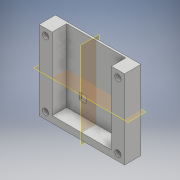
# Autodesk Inventor part: Case_Top_Partv1
Saved by Autodesk Inventor 2017 (Build 210142000, 142)
## iProperties
Created: 2020-01-23
Part Number: Case_Top_Partv1
Material: Generic
Document SubType Name: Modeling
Designer: Manny
Density: 1 g/cm^3
Appearance: Default
Author: Manny
Autodesk Inventor part; units mm, degrees
ref_plane "YZ Plane" through (0, 0, 0) normal (1, 0, 0) x (0, 1, 0)
ref_plane "XZ Plane" through (0, 0, 0) normal (0, 1, 0) x (-1, 0, 0)
ref_plane "XY Plane" through (0, 0, 0) normal (0, 0, 1) x (1, 0, 0)
sketch "Sketch1" plane through (0, 0, 0) normal (0, 1, 0) x (-1, 0, 0)
  line L0 (0, 0) -> (-130, 0)
  line L1 (-130, 0) -> (-130, -120)
  line L2 (-130, -120) -> (0, -120)
  line L3 (0, -120) -> (0, 0)
  dimension "d0" = 130
  dimension "d1" = 120
  constraints: 8 end point, 2 parallel, 1 horizontal, 1 perpendicular
  measures "d0" distance of L1.end L2.end
  measures "d1" distance of L0.end L1.end
extrude "Extrusion1" add sketch "Sketch1" along normal blind 25
sketch "Sketch2" plane through (0, 0, 0) normal (0, -1, 0) x (1, 0, 0)
  line L0 (110, -6.6572) -> (20, -6.6572)
  line L1 (20, -6.6572) -> (20, -110)
  line L2 (20, -110) -> (110, -110)
  line L3 (110, -110) -> (110, -6.6572)
  line L4 (0, -120) -> (0, 0) projected
  line L5 (0, 0) -> (130, 0) projected
  line L6 (130, -120) -> (0, -120) projected
  line L7 (130, 0) -> (130, -120) projected
  dimension "d5" = 6.6572
  dimension "d46" = 20
  dimension "d47" = 20
  dimension "d48" = 10
  constraints: 8 end point, 2 parallel, 1 horizontal, 1 perpendicular
  measures "d5" distance between parallel lines of L5 L0
  measures "d46" distance between parallel lines of L4 L1
  measures "d47" distance between parallel lines of L7 L3
  measures "d48" distance between parallel lines of L2 L6
extrude "Extrusion2" cut sketch "Sketch2" against normal blind 22 contours L3 L2 L1 L0
sketch "Sketch4" plane through (0, 22, 0) normal (0, -1, 0) x (1, 0, 0)
  line L0 (130, -120) -> (0, -120) projected
  line L1 (40, -90) -> (50, -90)
  line L2 (50, -90) -> (50, -80)
  line L3 (50, -80) -> (40, -80)
  line L4 (40, -80) -> (40, -90)
  line L5 (0, -120) -> (0, 0) projected
  line L6 (20, -110) -> (20, -6.6572) projected
  line L7 (110, -110) -> (20, -110) projected
  dimension "d42" = 10
  dimension "d43" = 10
  dimension "d49" = 20
  dimension "d50" = 20
  constraints: 8 end point, 2 parallel, 1 horizontal, 1 perpendicular
  measures "d42" distance of L1.start L1.end
  measures "d43" distance of L3.end L1.start
  measures "d49" distance between parallel lines of L4 L6
  measures "d50" distance between parallel lines of L1 L7
extrude "Extrusion3" cut sketch "Sketch4" against normal blind 22
sketch "Sketch5" plane through (0, 0, 0) normal (0, 0, 1) x (1, 0, 0)
  line L0 (20, 22) -> (110, 22)
  line L1 (110, 22) -> (110, 0)
  line L2 (110, 0) -> (20, 0)
  line L3 (20, 0) -> (20, 22)
  line L4 (0, 0) -> (0, 25) projected
  line L5 (130, 0) -> (130, 25) projected
  line L6 (0, 0) -> (130, 0) projected
  line L7 (130, 25) -> (0, 25) projected
  dimension "d13" = 20
  dimension "d14" = 20
  dimension "d15" = 0
  dimension "d16" = 3
  constraints: 8 end point, 2 parallel, 1 horizontal, 1 perpendicular
  measures "d13" distance between parallel lines of L4 L3
  measures "d14" distance between parallel lines of L5 L1
  measures "d15" distance between parallel lines of L6 L2
  measures "d16" distance between parallel lines of L7 L0
extrude "Extrusion4" cut sketch "Sketch5" against normal blind 22 contours L0 L1 L2 L3
sketch "Sketch10" plane through (0, 0, 0) normal (0, -1, 0) x (1, 0, 0)
  circle A0 centre (10, -10) radius 4.7625
  line L0 (0, 0) -> (20, 0) projected
  line L1 (0, -120) -> (0, 0) projected
  dimension "d51" = 10
  dimension "d52" = 10
  dimension "d53" = 9.525
  constraints: 1 centre point
  measures "d51" distance from line of L0 A0.centre
  measures "d52" distance from line of A0.centre L1
  measures "d53" diameter of A0
ref_plane "Work Plane3" through (65, 0, 0) normal (1, 0, 0) x (0, 0, -1)
ref_plane "Work Plane4" through (0, 25, -60) normal (0, 0, 1) x (1, 0, 0)
extrude "Extrusion7" cut sketch "Sketch10" against normal blind 25
mirror "Mirror4" about plane through (0, 25, -60) normal (0, 0, 1) of "Extrusion7"
mirror "Mirror5" about plane through (65, 0, 0) normal (1, 0, 0) of "Extrusion7", "Mirror4"
body "Solid1"
